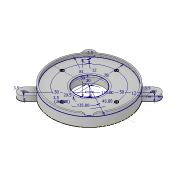
# Autodesk Inventor part: Lidar_circle
Saved by Autodesk Inventor 2019.4 (Build 234330000, 330)
## iProperties
Created: 2019-07-30
Part Number: Lidar_circle
Material: Generic
Document SubType Name: Modeling
Designer: leode
Density: 1 g/cm^3
Appearance: Default
Author: leode
Autodesk Inventor part; units mm, degrees
ref_plane "YZ Plane" through (0, 0, 0) normal (1, 0, 0) x (0, 1, 0)
ref_plane "XZ Plane" through (0, 0, 0) normal (0, 1, 0) x (-1, 0, 0)
ref_plane "XY Plane" through (0, 0, 0) normal (0, 0, 1) x (1, 0, 0)
sketch "Sketch1" plane through (0, 0, 0) normal (0, 1, 0) x (-1, 0, 0)
  circle A0 centre (0, 0) radius 39
  circle A1 centre (0, 0) radius 15
  circle A2 centre (0, 29.5) radius 1.75
  circle A3 centre (-29.5, 0) radius 1.75
  circle A4 centre (0, -29.5) radius 1.75
  circle A5 centre (29.5, 0) radius 1.75
  circle A6 centre (0, 0) radius 40.5
  line L0 (0, 0) -> (40.5, 0) construction
  line L1 (-31.0248, 26.0329) -> (-29.8757, 25.0687)
  line L2 (-25.0687, 29.8757) -> (-26.0329, 31.0248)
  dimension "d0" = 78
  dimension "d1" = 30
  dimension "d2" = 3.5
  dimension "d3" = 29.5
  dimension "d6" = 360
  dimension "d8" = 81
  constraints: 7 centre point, 6 end point, 4 coincident, 4 point on circle, 1 horizontal, 9 other
  measures "d0" diameter of A0
  measures "d1" diameter of A1
  measures "d2" diameter of A2
  measures "d3" distance of A1.centre A2.centre
  measures "d8" diameter of A6
extrude "Extrusion1" add sketch "Sketch1" along normal blind 3 contours A0 L2 A6 L1 picked at (-13.4532, -36.9622)
extrude "Extrusion2" add sketch "Sketch1" against normal blind 5
sketch "Sketch2" plane through (0, -5, 0) normal (0, -1, 0) x (1, 0, 0)
  circle A0 centre (0, 0) radius 15 projected
  circle A1 centre (-29.5, 0) radius 1.75 projected
  circle A2 centre (0, -29.5) radius 1.75 projected
  circle A3 centre (29.5, 0) radius 1.75 projected
  circle A4 centre (0, 29.5) radius 1.75 projected
  circle A5 centre (0, 0) radius 40.5 projected
  circle A6 centre (0, -29.5) radius 4
  circle A7 centre (-29.5, 0) radius 4
  circle A8 centre (0, 29.5) radius 4
  circle A9 centre (29.5, 0) radius 4
  dimension "d13" = 8
  dimension "d14" = 8
  dimension "d15" = 8
  dimension "d16" = 8
  constraints: 4 centre point, 4 coincident
  measures "d13" diameter of A6
  measures "d14" diameter of A7
  measures "d15" diameter of A8
  measures "d16" diameter of A9
extrude "Extrusion3" add sketch "Sketch2" along normal blind 5 contours A5
sketch "Sketch3" plane through (0, -10, 0) normal (0, -1, 0) x (1, 0, 0)
  line L0 (0, 0) -> (-28.6378, 28.6378)
  arc A0 (26.0329, 31.0248) -> (31.0248, 26.0329) centre (0, 0) ccw projected
  line L1 (0, 0) -> (40.5, 0) construction
  line L2 (0, 0) -> (-35.3553, 35.3553)
  line L3 (0, 0) -> (35.3553, -35.3553)
  line L4 (0, 0) -> (50, 0) construction
  line L5 (-35.3553, 35.3553) -> (35.3553, -35.3553) construction
  arc A1 (-31.1127, 39.598) -> (-39.598, 31.1127) centre (-35.3553, 35.3553) ccw
  arc A2 (31.1127, -39.598) -> (39.598, -31.1127) centre (35.3553, -35.3553) ccw
  circle A3 centre (0, 0) radius 40.5
  line L6 (-39.598, 31.1127) -> (-32.5645, 24.0792)
  line L7 (24.0792, -32.5645) -> (31.1127, -39.598)
  line L8 (39.598, -31.1127) -> (32.5645, -24.0792)
  line L9 (-24.0792, 32.5645) -> (-31.1127, 39.598)
  circle A4 centre (-35.3553, 35.3553) radius 1.75
  circle A5 centre (35.3553, -35.3553) radius 1.75
  line L10 (0, 0) -> (-35.3553, -35.3553) construction
  line L11 (-32.5645, -24.0792) -> (-39.598, -31.1127)
  line L12 (-31.1127, -39.598) -> (-24.0792, -32.5645)
  arc A6 (-39.598, -31.1127) -> (-31.1127, -39.598) centre (-35.3553, -35.3553) ccw
  line L13 (0, 0) -> (50, 0) construction
  circle A7 centre (-35.3553, -35.3553) radius 1.75
  point P0 (-17.6777, -17.6777)
  dimension "d22" = 135
  dimension "d26" = 50
  dimension "d27" = 50
  dimension "d28" = 45
  dimension "d29" = 12
  dimension "d30" = 3.5
  dimension "d31" = 3.5
  dimension "d34" = 50
  dimension "d35" = 135
  dimension "d36" = 12
  dimension "d37" = 3.5
  constraints: 32 end point, 13 point on circle, 10 tangent, 7 centre point, 5 parallel, 4 coincident, 3 equal length, 3 horizontal, 2 midpoint
  measures "d22" angle of L1 L0
  measures "d26" distance of L2.start L2.end
  measures "d27" distance of L2.start L3.end
  measures "d28" angle of L3 L4
  measures "d29" diameter of A2
  measures "d30" diameter of A4
  measures "d31" diameter of A5
  measures "d34" distance of L10.start L10.end
  measures "d35" angle of L10 L13
  measures "d36" diameter of A6
  measures "d37" diameter of A7
fillet "Fillet1" radius 2 4 edges at (25.5508, 0, 30.4503) (30.4503, 0, 25.5508) (25.5508, 3, 30.4503) (30.4503, 3, 25.5508)
fillet "Fillet3" radius 2 2 edges at (15, 0, 0) (-15, -10, 0)
extrude "Extrusion4" add sketch "Sketch3" against normal blind 5 contours A0 L6 A1 L9 | A0 L8 A2 L7 | A0 L12 A6 L11
body "Solid1"
